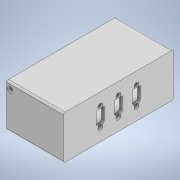
# Autodesk Inventor part: low_voltage_cover
Saved by Autodesk Inventor 2021.3 (Build 253353010, 353A)
## iProperties
Created: 2021-12-08
Part Number: low_voltage_cover
Material: Generic
Document SubType Name: Modeling
Designer: au504769
Density: 1 g/cm^3
Appearance: Default
Author: au504769
## iProperties of the stored document _3DPrint.ipt
Created: 2021-12-09
Part Number: _3DPrint
Material: Generic
Document SubType Name: Modeling
Designer: au504769
Density: 1 g/cm^3
Appearance: Default
Author: au504769
Autodesk Inventor part; units mm, degrees
ref_plane "YZ Plane" through (0, 0, 0) normal (1, 0, 0) x (0, 1, 0)
ref_plane "XZ Plane" through (0, 0, 0) normal (0, 1, 0) x (-1, 0, 0)
ref_plane "XY Plane" through (0, 0, 0) normal (0, 0, 1) x (1, 0, 0)
sketch "Sketch1" plane through (0, 0, 0) normal (1, 0, 0) x (0, 1, 0)
  line L0 (0, 0) -> (48, 0)
  line L1 (48, 0) -> (48, -122)
  line L2 (48, -122) -> (0, -122)
  line L3 (0, -122) -> (0, 0)
  line L4 (3, -3) -> (45, -3)
  line L5 (45, -3) -> (45, -119)
  line L6 (45, -119) -> (3, -119)
  line L7 (3, -119) -> (3, -3)
  line L8 (45, -6.2) -> (6.2, -6.2)
  line L9 (6.2, -6.2) -> (6.2, -115.8)
  line L10 (6.2, -115.8) -> (45, -115.8)
  line L11 (42, -6.2) -> (42, -115.8)
  line L12 (45, -3) -> (45, 0) construction
  line L13 (45, -3) -> (48, -3) construction
  line L14 (45, -119) -> (45, -122) construction
  line L15 (3, -3) -> (0, -3) construction
  line L16 (42, -6.2) -> (42, -3) construction
  line L17 (42, -59.8864) -> (45, -61) construction
  line L18 (6.2, -6.2) -> (3, -6.2) construction
  line L19 (42, -115.8) -> (42, -119) construction
  dimension "d0" = 116
  dimension "d1" = 42
  dimension "d2" = 3
  dimension "d3" = 3.2
  dimension "d5" = 3
  constraints: 40 end point, 12 perpendicular, 12 point on line, 6 equal length, 4 parallel, 3 horizontal, 1 midpoint
  measures "d0" distance between parallel lines of L6 L4
  measures "d1" distance between parallel lines of L7 L5
  measures "d2" distance between parallel lines of L0 L4
  measures "d3" distance between parallel lines of L4 L8
  measures "d5" distance between parallel lines of L5 L11
extrude "Extrusion1" add sketch "Sketch1" along normal blind 3 contours L0 L1 L2 L3 | L4 L5 L8 L9 L10 L6 L7 | L5 L10 L11 L8 | L11 L10 L9 L8
extrude "Extrusion2" add sketch "Sketch1" against normal blind 60
extrude "Extrusion3" add sketch "Sketch1" against normal blind 49 contours L5 L10 L11 L8
extrude "Extrusion4" add sketch "Sketch1" against normal blind 35 contours L4 L5 L8 L9 L10 L6 L7
sketch "Sketch2" plane through (-60, 3, -3) normal (0, 1, 0) x (1, 0, 0)
  line L0 (25, 3.2) -> (25, 112.8) projected
  line L1 (25, 6.5) -> (21.1, 6.5)
  arc A0 (21.1, 10.5) -> (21.1, 6.5) centre (21.1, 8.5) ccw
  line L2 (21.1, 10.5) -> (25, 10.5)
  line L3 (25, 10.5) -> (25, 6.5)
  line L4 (25, 0) -> (25, 116) projected
  line L5 (25, 109.5) -> (25, 105.5)
  line L6 (25, 105.5) -> (21.1, 105.5)
  arc A1 (21.1, 109.5) -> (21.1, 105.5) centre (21.1, 107.5) ccw
  line L7 (21.1, 109.5) -> (25, 109.5)
  line L8 (25, 105.5) -> (25, 10.5) construction
  line L9 (25, 109.5) -> (25, 112.8) construction
  line L10 (25, 6.5) -> (25, 3.2) construction
  point P0 (60, -3)
  point P1 (25, 109.5)
  dimension "d14" = 4
  dimension "d15" = 99
  dimension "d16" = 3.9
  constraints: 18 end point, 4 point on circle, 4 point on line, 4 tangent, 3 collinear, 3 equal length, 3 horizontal, 2 centre point, 2 perpendicular
  measures "d14" distance between parallel lines of L2 L1
  measures "d15" distance of A0.centre A1.centre
  measures "d16" distance from line of L0 A0.centre
extrude "Extrusion5" [suppressed]
sketch "Sketch10" plane through (3, 0, 0) normal (1, 0, 0) x (0, 0, -1)
  point P0 (0, 0)
sketch "Sketch11" plane through (3, 0, 0) normal (1, 0, 0) x (0, 0, -1)
  line L0 (59.75, 16) -> (62.25, 16)
  line L1 (65.25, 19) -> (65.25, 32)
  line L2 (65.25, 32) -> (56.75, 32)
  line L3 (56.75, 32) -> (56.75, 19)
  arc A0 (62.25, 16) -> (65.25, 19) centre (62.25, 19) ccw
  arc A1 (56.75, 19) -> (59.75, 16) centre (59.75, 19) ccw
  line L4 (0, 48) -> (0, 0) construction
  line L5 (122, 48) -> (0, 48) construction
  line L6 (61, 32) -> (0, 32) construction
  line L7 (61, 32) -> (122, 32) construction
  line L8 (122, 0) -> (122, 48) construction
  circle A2 centre (61, 34.3) radius 1.4 construction
  circle A3 centre (61, 13.7) radius 1.4 construction
  line L9 (61, 34.3) -> (61, 32) construction
  line L10 (61, 13.7) -> (61, 16) construction
  line L11 (61, 16) -> (61, 24) construction
  line L12 (61, 24) -> (61, 32) construction
  line L13 (61, 24) -> (61, 0) construction
  line L14 (0, 0) -> (122, 0) construction
  line L15 (61, 24) -> (61, 48) construction
  line L16 (0, 48) -> (122, 48) construction
  dimension "d69" = 16
  dimension "d70" = 8.5
  dimension "d113" = 20.6
  dimension "d115" = 2.8
  dimension "d116" = 3
  constraints: 24 end point, 5 collinear, 4 centre point, 4 midpoint, 4 point on circle, 4 point on line, 4 tangent, 3 coincident, 2 equal radius, 2 parallel, 2 perpendicular, 2 vertical, 1 horizontal, 1 vertical alignment
  measures "d69" distance between parallel lines of L2 L0
  measures "d70" distance between parallel lines of L1 L3
  measures "d113" distance of L9.start L10.start
  measures "d115" diameter of A2
  measures "d116" radius of A1
extrude "Extrusion8" cut sketch "Sketch11" against normal up to surface (3 mm away)
hole "Hole5" at (3, 34.3, -61) at (3, 13.7, -61) direction (-1, 0, 0) diameter 2.9 depth 3 tip angle 118 countersink diameter 5.5 countersink angle 90 clearance for "Countersunk Flat Head Screw DIN EN ISO 2009" size "M2.5" standard "DIN"
pattern_linear "Rectangular Pattern1" count 2 spacing 20 along (0, 0, -1) count 2 spacing 20 along (0, 0, 1) of "Extrusion8", "Hole5"
ref_plane "Work Plane2" through (-35, 42, -61) normal (0, 0, 1) x (1, 0, 0)
ref_plane "Work Plane3" through (-60, 22.5, -3) normal (0, 1, 0) x (1, 0, 0)
sketch "Sketch13" plane through (-35, 42, -61) normal (0, 0, 1) x (1, 0, 0)
  line L0 (35, -31.8) -> (27, -35.8)
  line L1 (27, -35.8) -> (35, -35.8) construction
  line L2 (35, -35.8) -> (35, -31.8) construction
  point P0 (35, -42)
  point P1 (35, 0)
  dimension "d87" = 4
  dimension "d88" = 8
  constraints: 6 end point, 1 coincident, 1 horizontal, 1 perpendicular
  measures "d87" distance of L1.end L0.start
  measures "d88" distance of L0.end L1.end
sketch "Sketch14" plane through (-60, 22.5, -3) normal (0, 1, 0) x (1, 0, 0)
  line L0 (60, 3.2) -> (35, 3.2) construction
  line L1 (35, 3.2) -> (60, 30.2)
  line L2 (60, 30.2) -> (60, 3.2) construction
  point P0 (60, -3)
  dimension "d101" = 27
  dimension "d102" = 25
  constraints: 6 end point, 1 horizontal, 1 vertical
  measures "d101" distance of L1.end L0.start
  measures "d102" distance of L0.start L0.end
extrude "Rib3" add sketch "Sketch14" along normal mid plane 2 rib yes fills toward (47.5367, 16.666) open curves L1
mirror "Mirror1" about plane through (-35, 42, -61) normal (0, 0, 1) of "Rib3"
feature "Rib1" [suppressed]
extrude "Rib2" add sketch "Sketch13" along normal mid plane 2 rib yes fills toward (31.0224, -33.8447) open curves L0
ref_plane "Work Plane5" through (-35, 24.1, -115.8) normal (0, 1, 0) x (1, 0, 0)
mirror "Mirror2" about plane through (-35, 24.1, -115.8) normal (0, 1, 0) of "Rib2"
fillet "Fillet1" radius 2 4 edges at (-17.5, 6.2, -115.8) (-47.5, 3, -119) (-17.5, 6.2, -6.2) (-47.5, 3, -3)
fillet "Fillet3" radius 2 4 edges at (-28.5, 48, -122) (-28.5, 0, -122) (-28.5, 0, 0) (-28.5, 48, 0)
fillet "Fillet4" radius 2 10 edges at (-12.5, 23.5, -6.2) (-12.5, 21.5, -6.2) (-4, 6.2, -60) (-4, 6.2, -62) (-12.5, 21.5, -115.8) (-12.5, 23.5, -115.8) (-17.5, 42, -115.8) (-17.5, 42, -6.2) (-4, 42, -60) (-4, 42, -62)
sketch "Sketch6" plane through (0, 0, 0) normal (0, 0, 1) x (1, 0, 0)
  line L0 (-35, 45) -> (-35, 5) projected
  line L1 (-35, 45) -> (-60, 45) projected
  point P0 (0, 0)
  point P1 (-56, 41)
  dimension "d42" = 4
  dimension "d43" = 21
  measures "d42" distance from line of point (-56, 41) L1
  measures "d43" distance from line of L0 point (-56, 41)
sketch "Sketch7" plane through (-60, 0, -2) normal (0, -1, 0) x (1, 0, 0)
  line L0 (22, -108.5) -> (22, -120) construction
  line L1 (63, -120) -> (0, -120) construction
  line L2 (22, -9.5) -> (22, 2) construction
  line L3 (0, 2) -> (63, 2) construction
  line L4 (25, -3) -> (25, -115) construction
  point P0 (60, 2)
  dimension "d33" = 99
  dimension "d34" = 3
  constraints: 4 end point, 3 point on line, 1 collinear, 1 vertical, 1 vertical alignment
  measures "d33" distance of L2.start L0.start
  measures "d34" distance from line of L4 L0.start
hole "Hole1" [suppressed]
hole "Hole2" at (-56, 41, 0) direction (0, 0, -1) diameter 3.4 depth 3 tip angle 118 countersink diameter 6.3 countersink angle 90 clearance for "Countersunk Flat Head Screw DIN EN ISO 2009" size "M3" standard "DIN"
sketch "Sketch9" plane through (3, 2, -122) normal (0, 0, -1) x (-1, 0, 0)
  circle A0 centre (59, 39) radius 3.15 projected
  point P0 (3, -2)
  constraints: 1 coincident
hole "Hole4" at (-56, 41, -122) direction (0, 0, 1) diameter 3.4 depth 3 tip angle 118 countersink diameter 6.3 countersink angle 90 clearance for "Countersunk Flat Head Screw DIN EN ISO 2009" size "M3" standard "DIN"
sketch "Sketch4" plane through (0, 0, 0) normal (0, 1, 0) x (-1, 0, 0)
  line L0 (-3, 0) -> (-3, -122) projected
  line L1 (60, 0) -> (-3, 0) projected
  line L2 (-3, -122) -> (31, -122)
  line L3 (31, -122) -> (31, 0)
  line L4 (31, 0) -> (-3, 0)
  line L5 (-3, 0) -> (-3, -122)
  point P0 (0, 0)
  point P1 (60, -122)
  dimension "d20" = 34
  constraints: 8 end point, 2 parallel, 1 horizontal, 1 perpendicular, 1 point on line
  measures "d20" distance between parallel lines of L0 L3
extrude "3D_print_test_cut_1" [suppressed]
sketch "Sketch12" plane through (0, 0, 0) normal (0, 1, 0) x (-1, 0, 0)
  line L0 (-3, -122) -> (60, -122) projected
  line L1 (-3, 0) -> (60, 0) projected
  line L2 (60, -122) -> (2, -122)
  line L3 (2, -122) -> (2, 0)
  line L4 (2, 0) -> (60, 0)
  line L5 (60, 0) -> (60, -122)
  line L6 (-3, -2) -> (-3, -120) projected
  point P0 (0, 0)
  dimension "d78" = 5
  constraints: 8 end point, 2 parallel, 1 horizontal, 1 perpendicular, 1 point on line
  measures "d78" distance between parallel lines of L6 L3
extrude "3D_print_test_cut_2" [suppressed]
ref_plane "Work Plane4" through (-56, 41, -145.4549) normal (-1, 0, 0) x (0, 0, 1)
body "Solid1"
